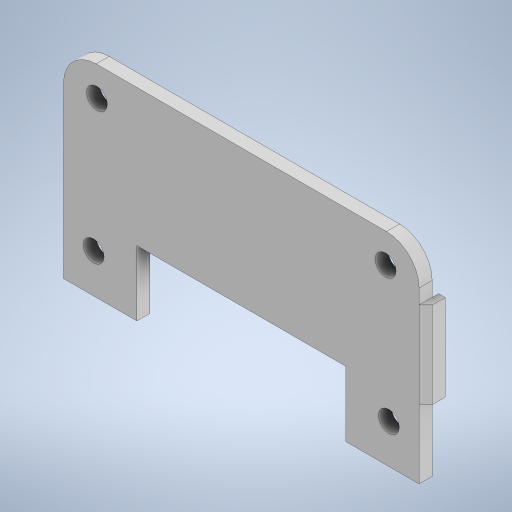
# Autodesk Inventor part: objímka_motorů
Saved by Autodesk Inventor 2023 (Build 270158000, 158)
## iProperties
Created: 2023-03-18
Part Number: objímka_motorů
Material: Všeobecné
Document SubType Name: Modeling
Designer: Simak
Density: 1 g/cm^3
Appearance: Výchozí
Author: Simak
Autodesk Inventor part; units mm, degrees
ref_plane "YZ Plane" through (0, 0, 0) normal (1, 0, 0) x (0, 1, 0)
ref_plane "XZ Plane" through (0, 0, 0) normal (0, 1, 0) x (-1, 0, 0)
ref_plane "XY Plane" through (0, 0, 0) normal (0, 0, 1) x (1, 0, 0)
sketch "Náčrt1" plane through (0, 0, 0) normal (0, 0, 1) x (1, 0, 0)
  line L0 (0, 0) -> (54.5, 0)
  line L1 (54.5, 0) -> (54.5, -31)
  line L2 (0, -31) -> (0, 0)
  line L3 (0, -7.25) -> (-1, -7.25)
  line L4 (-1, -7.25) -> (-1, -20.5)
  line L5 (-1, -20.5) -> (0, -20.5)
  line L6 (54.5, -7.25) -> (55.5, -7.25)
  line L7 (55.5, -7.25) -> (55.5, -20.5)
  line L8 (55.5, -20.5) -> (54.5, -20.5)
  line L9 (54.5, -31) -> (43.25, -31)
  line L10 (43.25, -31) -> (43.25, -21)
  line L11 (43.25, -21) -> (11.25, -21)
  line L12 (11.25, -21) -> (11.25, -31)
  line L13 (11.25, -31) -> (0, -31)
  dimension "d0" = 54.5
  dimension "d1" = 31
  dimension "d3" = 13.25
  dimension "d4" = 1
  dimension "d5" = 1
  dimension "d6" = 13.25
  dimension "d17" = 10
  dimension "d18" = 11.25
  dimension "d41" = 10.5
  dimension "d42" = 10.5
  constraints: 28 end point, 9 perpendicular, 5 point on line, 4 horizontal, 1 collinear, 1 parallel
  measures "d0" distance of L0.start L0.end
  measures "d1" distance of L0.end L1.end
  measures "d3" distance of L3.end L4.end
  measures "d4" distance of L3.start L3.end
  measures "d5" distance of L6.start L6.end
  measures "d6" distance of L6.end L7.end
  measures "d17" distance of L9.end L10.end
  measures "d18" distance of L1.end L9.end
  measures "d41" distance between parallel lines of L13 L5
  measures "d42" distance between parallel lines of L9 L8
extrude "Vysunutí1" add sketch "Náčrt1" along normal blind 2 contours L0 L1 L9 L10 L11 L12 L13 L2
extrude "Vysunutí2" add sketch "Náčrt1" along normal blind 2 and the other way blind 1 contours L2 L5 L4 L3 | L6 L7 L8 L1
chamfer "Zkosení1" distance 1 angle 45 2 edges at (-1, -13.875, 2) (55.5, -13.875, 2)
sketch "Náčrt2" plane through (0, 0, 2) normal (0, 0, 1) x (1, 0, 0)
  line L0 (43.25, -21) -> (43.25, -31) projected
  line L1 (54.5, -31) -> (54.5, -20.5) projected
  line L2 (43.25, -31) -> (54.5, -31) projected
  line L3 (49.375, -4.5) -> (54.5, -4.5) construction
  line L4 (54.5, -7.25) -> (54.5, 0) projected
  line L5 (5.125, -4.5) -> (0, -4.5) construction
  line L6 (0, 0) -> (0, -7.25) projected
  line L7 (54.5, 0) -> (0, 0) projected
  line L8 (0, -20.5) -> (0, -31) projected
  point P0 (49.875, -25)
  point P1 (4.625, -25)
  dimension "d20" = 6
  dimension "d28" = 44.25
  dimension "d31" = 6
  dimension "d50" = 4.625
  dimension "d51" = 4.5
  dimension "d52" = 4.625
  constraints: 4 end point, 3 point on line, 1 collinear, 1 horizontal, 1 parallel
  measures "d20" distance from line of L2 point (49.875, -25)
  measures "d28" distance of L5.start L3.start
  measures "d31" distance from line of point (4.625, -25) L2
  measures "d50" distance from line of L1 point (49.875, -25)
  measures "d51" distance from line of L7 L3.start
  measures "d52" distance from line of L8 point (4.625, -25)
hole "Díra2" at (49.875, -25, 2) at (49.375, -4.5, 2) at (5.125, -4.5, 2) at (4.625, -25, 2) direction (0, 0, -1) diameter 3.2 end through all
fillet "Zaoblení1" radius 5 2 edges at (0, 0, 1) (54.5, 0, 1)
ref_plane "Pracovní rovina1" through (9.25, -20.5, 0) normal (1, 0, 0) x (0, 0, -1)
sketch "Náčrt3" plane through (9.25, -20.5, 0) normal (1, 0, 0) x (0, 0, -1)
  line L0 (0, 0) -> (0, 13.25) projected
  line L1 (0, 1.5) -> (2.5, 1.5)
  line L2 (0, 11.75) -> (2.5, 11.75)
  line L3 (0, -10.5) -> (-2, -10.5) projected
  line L4 (0, 20.5) -> (-2, 20.5) projected
  arc A0 (2.5, 11.75) -> (2.5, 1.5) centre (6.5031, 6.625) ccw
  point P0 (0, 6.625)
  dimension "d43" = 10.25
  dimension "d44" = 2.5
  dimension "d45" = 12
  dimension "d47" = 6.5031
  constraints: 4 end point, 2 point on circle, 2 point on line, 1 centre point, 1 horizontal, 1 parallel, 1 perpendicular
  measures "d43" distance between parallel lines of L2 L1
  measures "d44" distance of L1.start L1.end
  measures "d45" distance between parallel lines of L1 L3
  measures "d47" radius of A0
extrude "Vysunutí3" add sketch "Náčrt3" along normal blind 14.75
ref_plane "Pracovní rovina2" through (27.25, -20.5, 0) normal (1, 0, 0) x (0, 0, -1)
mirror "Zrcadlit1" about plane through (27.25, -20.5, 0) normal (1, 0, 0) of "Vysunutí3"
